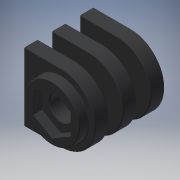
# Autodesk Inventor part: camera_bracket_female
Saved by Autodesk Inventor 2018 (Build 220112000, 112)
## iProperties
Created: 2018-06-20
Part Number: camera_bracket_female
Material: ABS Plastic
Document SubType Name: Modeling
Designer: car
Mass: 9.04679 g
Surface Area: 61.732 cm^2
Volume: 8.53471 cm^3
Density: 1.06 g/cm^3
Appearance: Carbon Fiber
iToolsLastSavedTime: 26-06-2018 09:38:27
iToolsLastSavedBy: car
iToolsMass: 0,000
LastSavedDate: 26-06-2018
LastSavedTime: 09:38:27
LastSavedBy: CAR
Reserved: False
Title: =<Part number>
Author: car
Autodesk Inventor part; units mm, degrees
ref_plane "YZ Plane" through (0, 0, 0) normal (1, 0, 0) x (0, 1, 0)
sketch "Sketch1" plane through (0, 0, 0) normal (0, 0, 1) x (1, 0, 0)
  circle A0 centre (0, 0) radius 7.5
  circle A1 centre (0, 0) radius 2.5
  line L0 (-7.5, -8) -> (7.5, -8)
  line L1 (7.5, -8) -> (7.5, 0)
  line L2 (-7.5, -8) -> (-7.5, 0)
  point P0 (0, -8)
  dimension "d2" = 15
  dimension "d3" = 5
  dimension "d6" = 8
  constraints: 6 end point, 2 centre point, 2 coincident, 2 point on circle, 2 tangent, 1 horizontal, 1 midpoint, 1 vertical alignment
  measures "d2" diameter of A0
  measures "d3" diameter of A1
  measures "d6" distance from line of L0 point (0, 0)
extrude "Extrusion2" add sketch "Sketch1" along normal mid plane 3
ref_plane "Work Plane1" through (0, 0, 4.6) normal (0, 0, 1) x (1, 0, 0)
ref_plane "Work Plane2" through (0, 0, -4.6) normal (0, 0, 1) x (1, 0, 0)
ref_plane "Work Plane3" through (0, 0, 7.6) normal (0, 0, 1) x (1, 0, 0)
ref_plane "Work Plane4" through (0, 0, -7.6) normal (0, 0, 1) x (1, 0, 0)
extrude "Extrusion3" add sketch "Sketch1" against normal up to surface (3 mm away) from surface at -4.6
extrude "Extrusion4" add sketch "Sketch1" along normal up to surface (3 mm away) from surface at 4.6
fillet "Fillet2" radius 0.2 10 edges at (0, 7.5, 7.6) (0, 7.5, -7.6) (0, 7.5, -4.6) (-7.5, -4, -1.5) (0, 7.5, -1.5) (7.5, -4, -1.5) (0, 7.5, 1.5) (-7.5, -4, 1.5) (0, 7.5, 4.6) (7.5, -4, 1.5)
sketch "Sketch4" plane through (0, 0, -7.6) normal (0, 0, -1) x (-1, 0, 0)
  circle A0 centre (0, 0) radius 2.5 projected
  line L0 (2.3671, 4.1) -> (4.7343, 0)
  line L1 (4.7343, 0) -> (2.3671, -4.1)
  line L2 (2.3671, -4.1) -> (-2.3671, -4.1)
  line L3 (-2.3671, -4.1) -> (-4.7343, 0)
  line L4 (-4.7343, 0) -> (-2.3671, 4.1)
  line L5 (-2.3671, 4.1) -> (2.3671, 4.1)
  circle A1 centre (0, 0) radius 6
  dimension "d28" = 8.2
  dimension "d29" = 12
  constraints: 12 end point, 2 coincident, 1 centre point, 13 other
  measures "d28" distance between parallel lines of L2 L5
  measures "d29" diameter of A1
extrude "Extrusion7" add sketch "Sketch4" along normal blind 2 contours A1
fillet "Fillet3" radius 0.2 2 edges at (6, 0, -7.6) (6, 0, -9.6)
chamfer "Chamfer1" distance 0.2 angle 45 6 edges at (-2.5, 0, -4.6) (-2.5, 0, -7.6) (-2.5, 0, -1.5) (-2.5, 0, 4.6) (-2.5, 0, 1.5) (-2.5, 0, 7.6)
body "Solid2"
